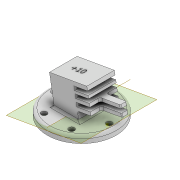
# Autodesk Inventor part: Plate_10
Saved by Autodesk Inventor 2022 (Build 260153000, 153)
## iProperties
Created: 2022-12-25
Part Number: Plate_10
Material: Generic
Document SubType Name: Modeling
Designer: dell
Density: 1 g/cm^3
Appearance: Default
Author: dell
Autodesk Inventor part; units mm, degrees
ref_plane "YZ Plane" through (0, 0, 0) normal (1, 0, 0) x (0, 1, 0)
ref_plane "XZ Plane" through (0, 0, 0) normal (0, 1, 0) x (-1, 0, 0)
ref_plane "XY Plane" through (0, 0, 0) normal (0, 0, 1) x (1, 0, 0)
sketch "Sketch1" plane through (0, 0, 0) normal (0, 1, 0) x (-1, 0, 0)
  circle A0 centre (0, 0) radius 50
  dimension "d0" = 100
  constraints: 1 centre point, 1 coincident
  measures "d0" diameter of A0
extrude "Extrusion1" add sketch "Sketch1" along normal blind 10
sketch "Sketch2" plane through (0, 10, 0) normal (0, 1, 0) x (1, 0, 0)
  circle A0 centre (-40, 0) radius 4.1
  point P0 (0, 0)
  dimension "d3" = 8.2
  dimension "d4" = 40
  constraints: 1 centre point
  measures "d3" diameter of A0
  measures "d4" distance of point (0, 0) A0.centre
extrude "Extrusion2" cut sketch "Sketch2" against normal blind 100
pattern_circular "Circular Pattern1" count 6 over 360 about axis through (0, 0, 0) along (0, 1, 0) of "Extrusion2"
ref_plane "Work Plane1" through (0, 10, -10) normal (0.1736482, -0.9848078, 0) x (0, 0, 1)
sketch "Sketch3" plane through (0, 10, 0) normal (-0.1736482, 0.9848078, 0) x (0.9848078, 0.1736482, 0)
  line L0 (-19.2365, 20) -> (15.7635, 20)
  line L1 (15.7635, 20) -> (15.7635, -20)
  line L2 (15.7635, -20) -> (-19.2365, -20)
  line L3 (-19.2365, -20) -> (-19.2365, 20)
  line L4 (-19.2365, 20) -> (15.7635, -20) construction
  line L5 (15.7635, 20) -> (-19.2365, -20) construction
  point P0 (-1.7365, 0)
  dimension "d10" = 35
  dimension "d11" = 40
  constraints: 12 end point, 2 midpoint, 2 parallel, 1 horizontal, 1 perpendicular
  measures "d10" distance of L1.end L2.end
  measures "d11" distance of L0.end L1.end
extrude "Extrusion3" add sketch "Sketch3" along normal blind 45
sketch "Sketch5" plane through (16.0067, 10, 20) normal (0.9848078, 0.1736482, 0) x (0, 0, -1)
  line L0 (0, 2.7795) -> (0, 47.7795) projected
  line L1 (40, 6.1714) -> (40, 47.7795) projected
  line L2 (0, 17.7795) -> (40, 17.7795)
  line L3 (40, 17.7795) -> (40, 12.7795)
  line L4 (40, 12.7795) -> (0, 12.7795)
  line L5 (0, 12.7795) -> (0, 17.7795)
  line L6 (0, 6.1714) -> (0, 47.7795) projected
  line L7 (0, 22.7795) -> (40, 22.7795)
  line L8 (40, 22.7795) -> (40, 27.7795)
  line L9 (40, 27.7795) -> (0, 27.7795)
  line L10 (0, 27.7795) -> (0, 22.7795)
  line L11 (40, 6.1714) -> (40, 47.7795) projected
  line L12 (0, 36.9795) -> (40, 36.9795)
  line L13 (40, 36.9795) -> (40, 32.7795)
  line L14 (40, 32.7795) -> (0, 32.7795)
  line L15 (0, 32.7795) -> (0, 36.9795)
  line L16 (0, 41.9795) -> (40, 41.9795)
  line L17 (40, 2.7795) -> (40, 47.7795) projected
  line L18 (0, 47.7795) -> (40, 47.7795) projected
  line L19 (0, 2.7795) -> (0, 47.7795) projected
  line L20 (0, 2.7795) -> (40, 2.7795) projected
  point P0 (20, -7.0685)
  point P1 (0, 0)
  point P2 (0, 12.7795)
  point P3 (0, 41.9795)
  point P4 (0, 32.7795)
  point P5 (40, 36.9795)
  point P6 (0, 36.9795)
  point P7 (0, 27.7795)
  point P8 (0, 22.7795)
  point P9 (40, 22.7795)
  dimension "d16" = 5
  dimension "d19" = 5
  dimension "d20" = 5
  dimension "d21" = 5
  dimension "d22" = 4.2
  dimension "d23" = 5
  dimension "d44" = 15
  constraints: 26 end point, 8 point on line, 6 parallel, 4 perpendicular, 3 horizontal
  measures "d16" distance between parallel lines of L2 L4
  measures "d19" distance between parallel lines of L7 L2
  measures "d20" distance between parallel lines of L7 L9
  measures "d21" distance between parallel lines of L9 L14
  measures "d22" distance between parallel lines of L14 L12
  measures "d23" distance between parallel lines of L12 L16
  measures "d44" distance between parallel lines of L20 L2
extrude "Extrusion4" add sketch "Sketch5" along normal blind 20 contours L0 L2 L1 L4 | L0 L9 L1 L7 | L0 L12 L1 L14 | L0 L18 L1 L16
sketch "Sketch7" plane through (35.7029, 13.473, 20) normal (0.9848078, 0.1736482, 0) x (0, 0, -1)
  point P0 (20, -7.0685)
sketch "Sketch6" plane through (35.7029, 13.473, 20) normal (0.9848078, 0.1736482, 0) x (0, 0, -1)
  line L0 (40, 12.7795) -> (40, 17.7795) projected
  line L1 (40, 17.7795) -> (0, 17.7795) projected
  line L2 (0, 17.7795) -> (0, 12.7795) projected
  line L3 (0, 12.7795) -> (40, 12.7795) projected
  line L4 (0, 27.7795) -> (0, 22.7795) projected
  line L5 (0, 22.7795) -> (40, 22.7795) projected
  line L6 (40, 22.7795) -> (40, 27.7795) projected
  line L7 (40, 27.7795) -> (0, 27.7795) projected
  line L8 (40, 27.7795) -> (0, 27.7795) projected
  line L9 (15.5, 27.7795) -> (24.5, 27.7795)
  line L10 (24.5, 27.7795) -> (24.5, 22.7795)
  line L11 (24.5, 22.7795) -> (15.5, 22.7795)
  line L12 (15.5, 22.7795) -> (15.5, 27.7795)
  line L13 (40, 17.7795) -> (0, 17.7795) projected
  line L14 (15.5, 17.7795) -> (24.5, 17.7795)
  line L15 (24.5, 17.7795) -> (24.5, 12.7795)
  line L16 (24.5, 12.7795) -> (15.5, 12.7795)
  line L17 (15.5, 12.7795) -> (15.5, 17.7795)
  line L18 (20, -31.1453) -> (20, 76.6153) projected
  point P0 (20, -7.0685)
  dimension "d24" = 9
  dimension "d25" = 9
  dimension "d26" = 4.5
  dimension "d27" = 4.5
  constraints: 16 end point, 4 parallel, 4 point on line, 2 horizontal, 2 perpendicular
  measures "d24" distance between parallel lines of L10 L12
  measures "d25" distance between parallel lines of L17 L15
  measures "d26" distance between parallel lines of L18 L12
  measures "d27" distance between parallel lines of L18 L17
extrude "Extrusion5" add sketch "Sketch6" along normal blind 30 contours L3 L18 L1 L15 | L3 L17 L1 L18 | L7 L18 L5 L12 | L7 L10 L5 L18
thicken "Thicken1" operation add thickness 0.2 both sides no extend neighbours yes toward (0.1736482, -0.9848078, 0) faces at (19.4847, 28.6671, -1.5)
thicken "Thicken2" operation add thickness 0.2 both sides no extend neighbours yes toward (-0.1736482, 0.9848078, 0) faces at (18.6165, 33.5911, 1.5)
thicken "Thicken3" operation add thickness 0.2 both sides no extend neighbours yes toward (0.1736482, -0.9848078, 0) faces at (17.7482, 38.5152, -1.5)
thicken "Thicken4" operation add thickness 0.2 both sides no extend neighbours yes toward (-0.1736482, 0.9848078, 0) faces at (23.4454, 44.5968, 6.6667)
thicken "Thicken5" operation add thickness 0.2 both sides no extend neighbours yes toward (0.1736482, -0.9848078, 0) faces at (22.716, 48.733, 6.6667)
thicken "Thicken6" operation add thickness 0.2 both sides no extend neighbours yes toward (-0.1736482, 0.9848078, 0) faces at (15.2824, 52.4994, 6.6667)
fillet "Fillet1" radius 3 8 edges at (-19.5332, 10, 0) (-9.7666, 10, -20) (-9.7666, 10, 20) (13.7876, 22.5854, 0) (33.067, 28.4219, -4.5) (31.3131, 38.3684, -4.5) (31.3131, 38.3684, 4.5) (33.067, 28.4219, 4.5)
chamfer "Chamfer1" distance 14 angle 45 1 edges at (0, 10, 0)
fillet "Fillet3" radius 10 1 edges at (14, 10, 0)
fillet "Fillet4" radius 4 1 edges at (50, 10, 0)
sketch "Sketch8" plane through (-7.8142, 54.3163, 0) normal (-0.1736482, 0.9848078, 0) x (0.9848078, 0.1736482, 0)
  line L0 (-6.9685, 4.6888) -> (10.8183, 4.6888) construction
  line L1 (10.8183, 4.6888) -> (10.8183, -13.2224) construction
  line L2 (10.8183, -13.2224) -> (-6.9685, -13.2224) construction
  line L3 (-6.9685, -13.2224) -> (-6.9685, 4.6888) construction
  line L4 (0.1952, -0.4004) -> (-2.5147, -0.4004)
  line L5 (-2.5147, -0.4004) -> (-2.5147, -3.1103)
  line L6 (-2.5147, -3.1103) -> (-3.4093, -3.1103)
  line L7 (-3.4093, -3.1103) -> (-3.4093, -0.4004)
  line L8 (-3.4093, -0.4004) -> (-6.1192, -0.4004)
  line L9 (-6.1192, -0.4004) -> (-6.1192, 0.4619)
  line L10 (-6.1192, 0.4619) -> (-3.4093, 0.4619)
  line L11 (-3.4093, 0.4619) -> (-3.4093, 3.1717)
  line L12 (-3.4093, 3.1717) -> (-2.5147, 3.1717)
  line L13 (-2.5147, 3.1717) -> (-2.5147, 0.4619)
  line L14 (-2.5147, 0.4619) -> (0.1952, 0.4619)
  line L15 (0.1952, 0.4619) -> (0.1952, -0.4004)
  line L16 (6.1531, -3.4733) -> (2.2503, -3.4733)
  line L17 (2.2503, -3.4733) -> (2.2503, -2.6565)
  line L18 (2.2503, -2.6565) -> (3.7025, -2.6565)
  line L19 (3.7025, -2.6565) -> (3.7025, 2.705)
  line L20 (3.7025, 2.705) -> (2.2503, 2.705)
  line L21 (2.2503, 2.705) -> (2.2503, 3.4375)
  spline S0 degree 2 poles (2.2503, 3.4375) (3.0736, 3.4375) (3.8516, 3.9043) (3.9035, 4.5526) knots 0 0 0 1 2 2 2
  line L22 (3.9035, 4.5526) -> (4.7333, 4.5526)
  line L23 (4.7333, 4.5526) -> (4.7333, -2.6565)
  line L24 (4.7333, -2.6565) -> (6.1531, -2.6565)
  line L25 (6.1531, -2.6565) -> (6.1531, -3.4733)
  spline S1 degree 2 poles (12.6036, 0.5267) (12.6036, -1.6257) (11.3524, -3.6419) (10.0493, -3.6419) knots 0 0 0 1 2 2 2
  spline S2 degree 2 poles (10.0493, -3.6419) (8.7268, -3.6419) (7.4886, -1.5868) (7.4886, 0.5202) knots 0 0 0 1 2 2 2
  spline S3 degree 2 poles (7.4886, 0.5202) (7.4886, 2.6855) (8.7398, 4.6888) (10.0493, 4.6888) knots 0 0 0 1 2 2 2
  spline S4 degree 2 poles (10.0493, 4.6888) (11.3654, 4.6888) (12.6036, 2.6142) (12.6036, 0.5267) knots 0 0 0 1 2 2 2
  spline S5 degree 2 poles (11.2292, -1.9109) (11.3848, -1.5154) (11.5145, -0.2966) (11.5145, 0.5267) knots 0 0 0 1 2 2 2
  spline S6 degree 2 poles (11.5145, 0.5267) (11.5145, 1.35) (11.3848, 2.5623) (11.2227, 2.9708) knots 0 0 0 1 2 2 2
  spline S7 degree 2 poles (11.2227, 2.9708) (11.0607, 3.3792) (10.4967, 3.8006) (10.0493, 3.8006) knots 0 0 0 1 2 2 2
  spline S8 degree 2 poles (10.0493, 3.8006) (9.602, 3.8006) (9.025, 3.3792) (8.8565, 2.9578) knots 0 0 0 1 2 2 2
  spline S9 degree 2 poles (8.8565, 2.9578) (8.6944, 2.5494) (8.5777, 1.3046) (8.5777, 0.5202) knots 0 0 0 1 2 2 2
  spline S10 degree 2 poles (8.5777, 0.5202) (8.5777, -0.3226) (8.6814, -1.4506) (8.85, -1.8915) knots 0 0 0 1 2 2 2
  spline S11 degree 2 poles (8.85, -1.8915) (9.0056, -2.3064) (9.5826, -2.7537) (10.0493, -2.7537) knots 0 0 0 1 2 2 2
  spline S12 degree 2 poles (10.0493, -2.7537) (10.4902, -2.7537) (11.0672, -2.3323) (11.2292, -1.9109) knots 0 0 0 1 2 2 2
  point P0 (-1.7365, 0)
  constraints: 2 other
extrude "Extrusion6" cut sketch "Sketch8" against normal blind 1
fillet "Fillet5" radius 1 4 edges at (62.6112, 33.6313, 4.5) (60.8573, 43.5779, 4.5) (60.8573, 43.5779, -4.5) (62.6112, 33.6313, -4.5)
equation "\"d26\" = 0.5 * d24"
equation "\"d27\" = 0.5 * d25"
body "Solid1"
